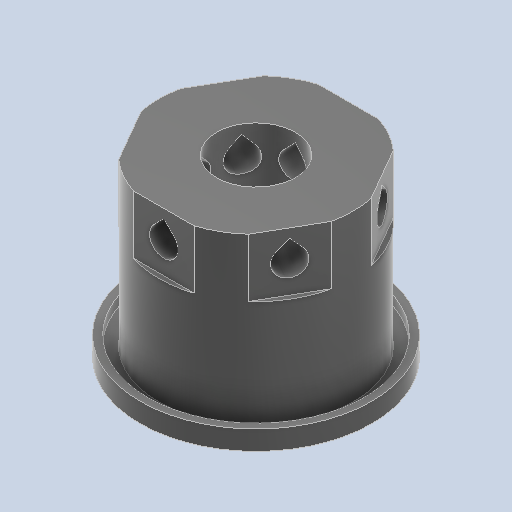
# Autodesk Inventor part: comutator_plastic
Saved by Autodesk Inventor 2025 (Build 290162000, 162)
## iProperties
Created: 2026-08-07
Part Number: comutator_plastic
Material: Ogólny
Document SubType Name: Modeling
Designer: zzapa
Density: 1 g/cm^3
Appearance: Gładki — czarny
Author: zzapa
Autodesk Inventor part; units mm, degrees
ref_plane "YZ Plane" through (0, 0, 0) normal (1, 0, 0) x (0, 1, 0)
ref_plane "XZ Plane" through (0, 0, 0) normal (0, 1, 0) x (-1, 0, 0)
ref_plane "XY Plane" through (0, 0, 0) normal (0, 0, 1) x (1, 0, 0)
sketch "Szkic1" plane through (0, 0, 0) normal (0, 1, 0) x (-1, 0, 0)
  circle A0 centre (0, 0) radius 10
  circle A1 centre (0, 0) radius 4.05
  dimension "d0" = 20
  dimension "d1" = 8.1
  constraints: 2 centre point, 2 coincident
  measures "d0" diameter of A0
  measures "d1" diameter of A1
extrude "Wyciągnięcie proste1" add sketch "Szkic1" along normal blind 17
sketch "Szkic2" plane through (0, 0, 0) normal (1, 0, 0) x (0, 1, 0)
  line L0 (17, -10) -> (17, 10) projected
  line L1 (0, -10) -> (0, 10) projected
  line L2 (17, -4.05) -> (0, -4.05) projected
  line L3 (0, -10) -> (17, -10) projected
  line L4 (17, -10) -> (11, -10)
  line L5 (11, -10) -> (11, -9.5)
  line L6 (11, -9.5) -> (17, -9.5)
  line L7 (17, -9.5) -> (17, -10)
  point P0 (0, 0)
  point P1 (11, -10)
  dimension "d9" = 0.5
  dimension "d10" = 6
  constraints: 8 end point, 2 collinear, 2 parallel, 1 horizontal, 1 perpendicular
  measures "d9" distance of L4.end L5.end
  measures "d10" distance of L5.end L6.end
extrude "Wyciągnięcie proste2" cut sketch "Szkic2" along normal through all both and the other way through all contours L3 L5 L6 L0
pattern_circular "Szyk kołowy1" count 6 over 360 about axis through (0, -10, 0) along (0, 1, 0) of "Wyciągnięcie proste2"
sketch "Szkic3" plane through (3.1225, 17, -9.5) normal (0, 0, -1) x (-1, 0, 0)
  line L0 (6.245, 0) -> (6.245, -6) projected
  line L1 (0, 0) -> (6.245, 0) projected
  line L2 (0, -6) -> (0, 0) projected
  line L3 (0, -6) -> (6.245, -6) projected
  line L4 (0, 0) -> (6.245, 0) projected
  line L5 (0, -6) -> (6.245, -6) projected
  line L6 (3.1225, -6) -> (3.1225, 0)
  point P0 (3.1225, -17)
  point P1 (3.1225, -3)
  dimension "d21" = 3
  constraints: 3 midpoint, 2 end point
  measures "d21" distance from line of L1 point (3.122, -3)
hole "Otwór1" at (0, 14, -9.5) direction (0, 0, 1) diameter 2.9 depth 9.5
pattern_circular "Szyk kołowy2" count 6 over 360 about axis through (0, -10, 0) along (0, 1, 0) of "Otwór1"
sketch "Szkic4" plane through (0, 17, 0) normal (0, 1, 0) x (1, 0, 0)
  arc A0 (3.1225, -9.5) -> (6.666, -7.4542) centre (0, 0) ccw projected
  arc A1 (9.7885, -2.0458) -> (9.7885, 2.0458) centre (0, 0) ccw projected
  arc A2 (-6.666, -7.4542) -> (-3.1225, -9.5) centre (0, 0) ccw projected
  arc A3 (-9.7885, 2.0458) -> (-9.7885, -2.0458) centre (0, 0) ccw projected
  arc A4 (-3.1225, 9.5) -> (-6.666, 7.4542) centre (0, 0) ccw projected
  arc A5 (6.666, 7.4542) -> (3.1225, 9.5) centre (0, 0) ccw projected
  line L0 (8.1209, -14.0659) -> (-8.8865, 15.3918)
  line L1 (9.1342, 15.8208) -> (-8.7747, -15.1982)
  line L2 (-25.8919, 0) -> (19.9485, 0)
  circle A6 centre (0, 0) radius 11
  circle A7 centre (0, 0) radius 11.5
  circle A8 centre (0, 0) radius 12
  line L3 (-26.4275, -39.1803) -> (-43.4349, -9.7227)
  line L4 (-25.4142, -9.2936) -> (-43.3231, -40.3126)
  line L5 (-60.4403, -25.1145) -> (-14.5998, -25.1145)
  circle A9 centre (-34.5484, -25.1145) radius 11
  circle A10 centre (-34.5484, -25.1145) radius 11.5
  circle A11 centre (-34.5484, -25.1145) radius 12
  point P0 (5, -8.6603)
  point P1 (-5, 8.6603)
  point P2 (-10, 0)
  point P3 (10, 0)
  point P4 (5, 8.6603)
  point P5 (-5, -8.6603)
  point P6 (-29.5484, -33.7747)
  point P7 (-39.5484, -16.4542)
  point P8 (-44.5484, -25.1145)
  point P9 (-24.5484, -25.1145)
  point P10 (-29.5484, -16.4542)
  point P11 (-39.5484, -33.7747)
  point P12 (5.5, -9.5263)
  point P13 (11, 0)
  dimension "d22" = 22
  dimension "d23" = 23
  dimension "d24" = 24
  dimension "d25" = 22
  dimension "d26" = 23
  dimension "d27" = 24
  constraints: 14 point on line, 12 end point, 8 point on circle, 6 centre point, 5 coincident, 2 horizontal
  measures "d22" diameter of A6
  measures "d23" diameter of A7
  measures "d24" diameter of A8
  measures "d25" diameter of A9
  measures "d26" diameter of A10
  measures "d27" diameter of A11
sketch "Szkic5" plane through (0, 0, 0) normal (1, 0, 0) x (0, 1, 0)
  line L0 (-1, 11.9) -> (0, 11.9)
  line L1 (0, 11.9) -> (0, 4.05)
  line L2 (0, 4.05) -> (-1, 4.05)
  line L3 (-1, 4.05) -> (-1, 11.9)
  line L4 (0, -10) -> (0, 10) projected
  line L5 (0, 10) -> (11, 10) projected
  line L6 (1, 11.9) -> (0, 11.9)
  line L7 (0, 11.9) -> (0, 11.15)
  line L8 (0, 11.15) -> (1, 11.15)
  line L9 (1, 11.15) -> (1, 11.9)
  line L10 (17, 4.05) -> (17, -4.05) projected
  line L11 (0, 4.05) -> (0, -4.05) projected
  line L12 (-4.6, 0) -> (20.6, 0) projected
  point P0 (0, 0)
  point P1 (14, 3.7815)
  point P2 (14, -3.7815)
  point P3 (0, 0)
  point P4 (0, 11.9)
  point P5 (0, 11.15)
  dimension "d28" = 11.9
  dimension "d29" = 1
  dimension "d30" = 11.15
  dimension "d31" = 1
  constraints: 16 end point, 4 parallel, 3 collinear, 2 horizontal, 2 perpendicular, 1 midpoint, 1 point on line, 4 other
  measures "d28" distance from line of point (0, 0) L0
  measures "d29" distance of L1.end L2.end
  measures "d30" distance from line of point (0, 0) L8
  measures "d31" distance between parallel lines of L1 L9
revolve "Obrót1" add sketch "Szkic5" angle 360 about axis through (0, -10, 0) along (0, 1, 0)
sketch "Szkic6" plane through (-6.666, 11, 7.4542) normal (-0.8660254, 0, 0.5) x (0.5, 0, 0.8660254)
  circle A0 centre (-3.1225, 3) radius 1.45 projected
  line L0 (-6.245, 6) -> (0, 6) projected
  line L1 (-6.245, 0) -> (0, 0) projected
  line L2 (-3.1225, 3) -> (-3.1225, 6)
  line L3 (-2.0972, 4.0253) -> (-3.1225, 5.0506)
  line L4 (-4.1478, 4.0253) -> (-3.1225, 5.0506)
  point P0 (-3.1225, -11)
  dimension "d33" = 90
  constraints: 6 end point, 1 coincident, 1 midpoint, 1 point on line, 1 symmetric about line, 3 other
  measures "d33" angle of L3 L4
extrude "Wyciągnięcie proste3" cut sketch "Szkic6" against normal up to surface contours A0 L2 L3 | L4 L2 A0 round surface about axis through (0, 0, 0) along (0, 1, 0) radius 4.05 far side no
pattern_circular "Szyk kołowy3" count 6 over 360 about axis through (0, -10, 0) along (0, 1, 0) of "Wyciągnięcie proste3"
equation "\"d0\" = commutator_plastic_D"
equation "\"d1\" = commutator_plastic_shaft_d"
equation "\"d2\" = commutator_plastic_h"
equation "\"d9\" = commutator_plastic_insert_cut_deepness"
equation "\"d10\" = commutator_plastic_insert_cut_length"
equation "\"d21\" = commutator_plastic_insert_pos"
equation "\"d11\" = insert_m2_d"
equation "\"d28\" = commutator_plastic_back_plate_lock_r"
equation "\"d29\" = commutator_plastic_back_plate_lock_h"
equation "\"d30\" = commutator_plastic_back_plate_hook_in_r"
equation "\"d31\" = commutator_plastic_back_plate_hook_h"
equation "\"insert_m2_d\" = 2.9"
equation "\"insert_m2_h\" = 7"
equation "\"insert_m2_corner\" = 0.5"
equation "\"insert_m2_pocket_d\" = 2.6"
equation "\"insert_m2_pocket_D\" = 4.5"
equation "\"insert_m2_pocket_nut_h\" = 1.5"
equation "\"stator_r_out\" = 30.15"
equation "\"stator_out_d\" = 3.2"
equation "\"stator_h\" = 45"
equation "\"mag_size_x\" = 7"
equation "\"mag_size_y\" = 3"
equation "\"mag_corner_r\" = 0.4"
equation "\"magnet_ring_r\" = 26.95"
equation "\"magnet_ring_d\" = 3.3"
equation "\"magnet_ring_h\" = 36"
equation "\"magnet_ring_pocket_mag_size_x\" = 7.1"
equation "\"magnet_ring_pocket_mag_size_y\" = 3.1"
equation "\"magnet_ring_pocket_mag_size_z\" = 10.1"
equation "\"magnet_ring_pocket_radial_cut\" = 1.4"
equation "\"casing_d\" = 3"
equation "\"casing_r_in\" = 30.15"
equation "\"rotor_out_r\" = 22.5"
equation "\"rotor_coil_groove_in_r\" = 17"
equation "\"rotor_coil_groove_ang\" = 18deg"
equation "\"rotor_core_r\" = 14.97"
equation "\"rotor_coil_groove_in_correction_r\" = 18"
equation "\"rotor_plastic_h\" = 32"
equation "\"rotor_teeth_d\" = 1.5"
equation "\"rotor_plastic_insert_r\" = 37"
equation "\"shaft_d\" = 8"
equation "\"shaft_lock_1_d\" = 8.1"
equation "\"shaft_lock_1_D\" = 44"
equation "\"shaft_lock_1_h1\" = 3.5"
equation "\"shaft_lock_1_corner\" = 2"
equation "\"shaft_lock_1_rotor_insert_grove_d_in\" = 36"
equation "\"shaft_lock_1_rotor_insert_grove_width_out\" = 5.5"
equation "\"shaft_lock_1_rotor_insert_grove_width_in\" = 7.6"
equation "\"shaft_lock_1_rotor_insert_r\" = 37"
equation "\"shaft_lock_1_shaft_insert_axial_cut_out_width\" = 12"
equation "\"shaft_lock_1_shaft_insert_axial_cut_in_width\" = 5.4"
equation "\"shaft_lock_1_shaft_insert_pos\" = 2.5"
equation "\"shaft_lock_1_shaft_insert_corner\" = 2"
equation "\"shaft_lock_1_shaft_insert_corner_finish\" = 0.5"
equation "\"shaft_lock_2_d\" = 8.1"
equation "\"shaft_lock_2_D\" = 44"
equation "\"shaft_lock_2_h1\" = 3.5"
equation "\"shaft_lock_2_corner\" = 2"
equation "\"shaft_lock_2_rotor_insert_grove_d_in\" = 36"
equation "\"shaft_lock_2_rotor_insert_grove_width_out\" = 5.5"
equation "\"shaft_lock_2_rotor_insert_grove_width_in\" = 7.6"
equation "\"shaft_lock_2_rotor_insert_r\" = 37"
equation "\"shaft_lock_2_shaft_insert_axial_cut_out_width\" = 12"
equation "\"shaft_lock_2_shaft_insert_axial_cut_in_width\" = 5.4"
equation "\"shaft_lock_2_shaft_insert_pos\" = 2.5"
equation "\"shaft_lock_2_shaft_insert_corner\" = 2"
equation "\"shaft_lock_2_shaft_insert_corner_finish\" = 0.5"
equation "\"commutator_plastic_D\" = 20"
equation "\"commutator_plastic_h\" = 17"
equation "\"commutator_plate_D\" = 22"
equation "\"commutator_plate_d\" = 1"
equation "\"commutator_plate_ang\" = 55deg"
equation "\"commutator_plate_h\" = 17"
equation "\"commutator_plastic_shaft_d\" = 8.1"
equation "\"commutator_plastic_insert_cut_deepness\" = 0.5"
equation "\"commutator_plastic_insert_cut_length\" = 6"
equation "\"commutator_plastic_insert_pos\" = 3"
equation "\"commutator_plate_insert_pos\" = 3"
equation "\"casing_lock_hole_r\" = 14.25"
equation "\"casing_lock_h\" = 8"
equation "\"casing_stator_fix_r\" = 23"
equation "\"casing_stator_fix_h\" = 6"
equation "\"magnet_ring_insert_part_lengthen\" = 8"
equation "\"casing_sidebar_length\" = 3"
equation "\"casing_vent_hole_length\" = 4"
equation "\"casing_vent_hole_width\" = 6"
equation "\"sleeve_cup_r\" = 22"
equation "\"sleeve_cup_h\" = 4.5"
equation "\"sleeve_h\" = 7"
equation "\"sleeve_d\" = 3"
equation "\"sleeve_in_r\" = 11.1"
equation "\"casing_head_insert_r\" = 19"
equation "\"sleeve_head_insert_r\" = 19"
equation "\"magnet_ring_insert_part_radius_cut\" = 0.17"
equation "\"magnet_ring_insert_part_axial_flat_cut\" = 0.17"
equation "\"magnet_ring_insert_pos\" = 4"
equation "\"casing_radial_stator_insert_pos\" = 18.1"
equation "\"stator_radial_screw_d\" = 4"
equation "\"stator_radial_screw_pos\" = 4"
equation "\"rotor_sleeve_out_D\" = 10.5"
equation "\"rotor_sleeve_in_D\" = 8.15"
equation "\"rotor_sleeve_h\" = 32"
equation "\"carbon_brush_batt_h\" = 8"
equation "\"carbon_brush_batt_d\" = 4"
equation "\"brush_cart_outer_holder_width\" = 5.5"
equation "\"brush_cart_outer_holder_arc_r\" = 33.15"
equation "\"brush_cart_outer_holder_arc_pos\" = 1.5"
equation "\"casing_cart_hole_corner\" = 1"
equation "\"casing_cart_hole_width\" = 2.6"
equation "\"casing_cart_hole_ang\" = 90deg"
equation "\"brush_holder_batt_arc_r\" = 30.15"
equation "\"brush_holder_batt_width\" = 16"
equation "\"brush_holder_batt_insert_flat_length\" = 6"
equation "\"brush_holder_batt_insert_flat_depth\" = 6"
equation "\"brush_holder_batt_insert_flat_width\" = 2"
equation "\"brush_holder_batt_brush_hole_d\" = 4.5"
equation "\"casing_backsleeve_insert_pos\" = 4.9"
equation "\"casing_cart_hole_pos\" = 17"
equation "\"casing_sleeve_cut_d\" = 46"
equation "\"casing_sleeve_cut_h\" = 4"
equation "\"name_plate_D\" = 45"
equation "\"name_plate_d\" = 28"
equation "\"name_plate_insert_r\" = 19"
equation "\"sleeve_bearing_material_lock_h\" = 2"
equation "\"back_sleeve_D\" = 66"
equation "\"back_sleeve_d\" = 22.2"
equation "\"back_sleeve_h\" = 5"
equation "\"commutator_back_plate_lock_h\" = 2"
equation "\"commutator_back_plate_lock_r\" = 23"
equation "\"commutator_plastic_back_plate_lock_r\" = 11.9"
equation "\"commutator_plastic_back_plate_lock_h\" = 1"
equation "\"commutator_plastic_back_plate_hook_h\" = 1"
equation "\"commutator_plastic_back_plate_hook_in_r\" = 11.15"
